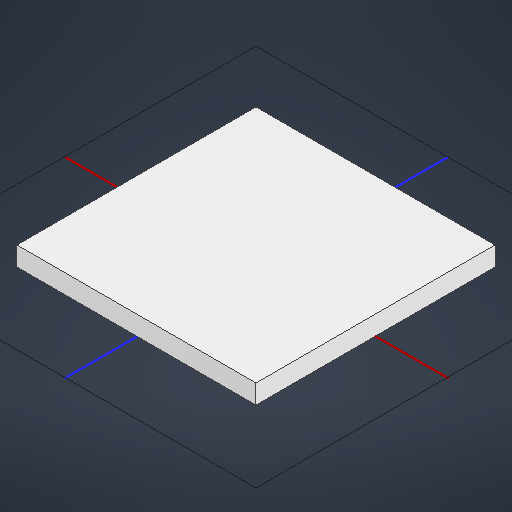
# Autodesk Inventor part: White Square
Saved by Autodesk Inventor 2026 (Build 300175000, 175)
## iProperties
Created: 2025-04-18
Part Number: White Square
Material: ABS Plastic
Document SubType Name: Modeling
Designer: ckyiu
Density: 1.06 g/cm^3
Appearance: Smooth - White
Author: ckyiu
Autodesk Inventor part; units mm, degrees
ref_plane "YZ Plane" through (0, 0, 0) normal (1, 0, 0) x (0, 1, 0)
ref_plane "XZ Plane" through (0, 0, 0) normal (0, 1, 0) x (-1, 0, 0)
ref_plane "XY Plane" through (0, 0, 0) normal (0, 0, 1) x (1, 0, 0)
sketch "Sketch1" plane through (0, 0, 0) normal (0, 1, 0) x (-1, 0, 0)
  line L0 (12.5, -12.5) -> (-12.5, -12.5)
  line L1 (-12.5, -12.5) -> (-12.5, 12.5)
  line L2 (-12.5, 12.5) -> (12.5, 12.5)
  line L3 (12.5, 12.5) -> (12.5, -12.5)
  line L4 (12.5, -12.5) -> (-12.5, 12.5) construction
  line L5 (-12.5, -12.5) -> (12.5, 12.5) construction
  point P0 (0, 0)
  dimension "d0" = 25
  dimension "d1" = 25
  constraints: 12 end point, 2 midpoint, 2 parallel, 1 horizontal, 1 perpendicular
  measures "d0" distance of L1.end L2.end
  measures "d1" distance of L0.end L1.end
extrude "Extrusion1" add sketch "Sketch1" along normal blind 2
sketch "Sketch2" plane through (0, 0, 0) normal (0, -1, 0) x (1, 0, 0)
  line L0 (-12.5, -12.5) -> (-12.5, 12.5) construction
  line L1 (-12.5, 12.5) -> (0, 0) construction
  line L2 (-12.5, 0) -> (0, 12.5) construction
  line L3 (-12.5, 12.5) -> (12.5, 12.5) construction
  circle A0 centre (-6.25, 6.25) radius 1.5
  line L4 (0, 12.5) -> (0, 0) construction
  line L5 (0, 0) -> (-12.5, 0) construction
  circle A1 centre (6.25, 6.25) radius 1.5
  circle A2 centre (-6.25, -6.25) radius 1.5
  circle A3 centre (6.25, -6.25) radius 1.5
  dimension "d4" = 3
  constraints: 8 end point, 4 centre point, 4 midpoint, 3 symmetric about line, 2 perpendicular, 3 other
  measures "d4" diameter of A0
extrude "Extrusion2" cut sketch "Sketch2" against normal blind 1
equation "\"d0\" = 0.125 * chessboard_length"
equation "\"d1\" = 0.125 * chessboard_width"
equation "\"d2\" = square_thickness"
equation "\"d4\" = peg_diameter"
equation "\"d5\" = peg_height"
equation "\"square_thickness\" = 2"
equation "\"chessboard_length\" = 200"
equation "\"chessboard_width\" = 200"
equation "\"peg_diameter\" = 3"
equation "\"peg_height\" = 1"
body "Solid1"
